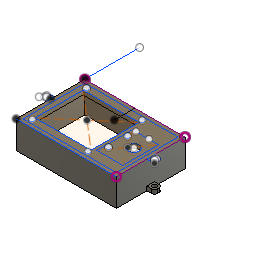
Suporte LCD Nokia 5110 e Botao de Encoder v3 (Autodesk Fusion 360 design; units mm, degrees)
Autodesk Fusion 360 part; units mm, degrees
sketch "Sketch1" plane through (0, 0, 0) normal (0, 1, 0) x (1, 0, 0)
  line L0 (72, -50) -> (-1, -50)
  line L1 (1.5, -2.5) -> (69.5, -2.5)
  line L2 (69.5, -47.5) -> (1.5, -47.5)
  circle A0 centre (5.5, -5.25) radius 1.5
  circle A1 centre (5.5, -44.75) radius 1.5
  circle A2 centre (46, -5.25) radius 1.5
  circle A3 centre (46, -44.75) radius 1.5
  line L3 (46, -7.5) -> (5.25, -7.5)
  line L4 (5.25, -7.5) -> (5.25, -42.5)
  line L5 (5.25, -42.5) -> (46, -42.5)
  line L6 (46, -42.5) -> (46, -7.5)
  line L7 (46, -7.5) -> (5.25, -42.5) construction
  line L8 (5.25, -7.5) -> (46, -42.5) construction
  line L9 (72, 0) -> (-1, 0)
  line L10 (-1, 39.9342) -> (-1, -50)
  line L11 (1.5, -47.5) -> (1.5, -2.5)
  line L12 (67.25, -14.5) -> (48.25, -14.5)
  line L13 (48.25, -14.5) -> (48.25, -40.5)
  line L14 (48.25, -40.5) -> (67.25, -40.5)
  line L15 (67.25, -40.5) -> (67.25, -14.5)
  line L16 (67.25, -14.5) -> (48.25, -40.5) construction
  line L17 (48.25, -14.5) -> (67.25, -40.5) construction
  line L18 (67.25, -14.5) -> (60.25, -14.5)
  line L19 (69.5, -2.5) -> (69.5, -47.5)
  line L20 (72, 0) -> (72, -50)
  circle A4 centre (60.25, -25.5) radius 3.875
  line L21 (48.25, -14.5) -> (50.75, -14.5)
  circle A5 centre (50.75, -20.5) radius 1.5
  circle A6 centre (50.75, -34.5) radius 1.5
  point P0 (25.625, -25)
  point P1 (57.75, -27.5)
  dimension "d10" = 3
  dimension "d12" = 35
  dimension "d15" = 19
  dimension "d19" = 26
  dimension "d20" = 2.5
  dimension "d21" = 40.75
  dimension "d22" = 4
  dimension "d30" = 7.75
  dimension "d31" = 2.5
  dimension "d32" = 6
  dimension "d34" = 3
  dimension "d35" = 3
  dimension "d36" = 7
  dimension "d37" = 11
  constraint horizontal L9
  constraint horizontal L0
  constraint perpendicular L3 L4
  constraint parallel L3 L5
  constraint parallel L4 L6
  constraint horizontal L3
  constraint coincident L7 P0
  constraint coincident L8 P0
  constraint perpendicular L9 L10
  constraint parallel L1 L9
  constraint parallel L0 L2
  constraint perpendicular L12 L13
  constraint parallel L12 L14
  constraint parallel L13 L15
  constraint horizontal L12
  constraint coincident L16 P1
  constraint coincident L17 P1
  constraint horizontal L18
  constraint coincident L9.end L10
  constraint perpendicular L13 L21
  measures "d10" diameter of A3
  measures "d12" distance of L3.end L4.end
  measures "d15" distance of L13.end L14.end
  measures "d19" distance of L12.start L14.end
  measures "d20" distance of L10 L11
  measures "d21" distance of L3.start L3.end
  measures "d22" distance of A0.centre L11
  measures "d30" diameter of A4
  measures "d31" distance of L12.end L21.end
  measures "d32" distance of L21.end A5.centre
  measures "d34" diameter of A5
  measures "d35" diameter of A6
  measures "d36" distance of L15 A4.centre
  measures "d37" distance of L12 A4.centre
extrude "Extrude1" add sketch "Sketch1" against normal blind 3 contours L1 L2 L11 L19 | L12 L13 L14 L15 L18 L21
extrude "Extrude2" add sketch "Sketch1" against normal blind 20 contours L0 L9 L10 L20
sketch "Sketch2" plane through (0, 0, 0) normal (0, 1, 0) x (1, 0, 0)
  line L0 (72, 0) -> (72, -50)
  line L1 (72, -25) -> (72, -27.75)
  line L2 (72, -27.75) -> (75.5, -27.75)
  line L3 (77.5, -25.75) -> (77.5, -24.25)
  line L4 (75.5, -22.25) -> (72, -22.25)
  line L5 (72, -22.25) -> (72, -27.75)
  circle A0 centre (74.75, -25) radius 1.5
  line L6 (72, 0) -> (-1, 0)
  line L7 (35.5, 0) -> (35.5, -15)
  arc A1 (77.5, -24.25) -> (75.5, -22.25) centre (75.5, -24.25) ccw
  arc A2 (75.5, -27.75) -> (77.5, -25.75) centre (75.5, -25.75) ccw
  circle A3 centre (-3.75, -25) radius 1.5
  arc A4 (-6.5, -25.75) -> (-4.5, -27.75) centre (-4.5, -25.75) ccw
  arc A5 (-4.5, -22.25) -> (-6.5, -24.25) centre (-4.5, -24.25) ccw
  line L8 (-1, -22.25) -> (-1, -27.75)
  line L9 (-4.5, -22.25) -> (-1, -22.25)
  line L10 (-6.5, -25.75) -> (-6.5, -24.25)
  line L11 (-1, -27.75) -> (-4.5, -27.75)
  line L12 (-1, 0) -> (-1, -50)
  line L13 (-1, -25) -> (-1, -27.75)
  point P0 (77.5, -27.75)
  point P1 (-6.5, -27.75)
  dimension "d45" = 5.5
  dimension "d46" = 5.5
  dimension "d47" = 3
  dimension "d48" = 15
  dimension "d49" = 2
  dimension "d50" = 2
  constraint midpoint L0 L1.start
  constraint horizontal L2
  constraint vertical L3
  constraint horizontal L4
  constraint vertical L5
  constraint midpoint L6 L7.start
  constraint perpendicular L6 L7
  constraint tangent L3 A1
  constraint tangent L4 A1
  constraint coincident P0 L3
  constraint coincident P0 L2
  constraint tangent L3 A2
  constraint tangent L2 A2
  constraint symmetric L0.start L7 L6.end
  constraint symmetric L0.end L7 L12.end
  constraint symmetric L1.start L7 L13.start
  constraint symmetric L1.end L7 L8.end
  constraint symmetric P0 L7 P1
  constraint symmetric L4.end L7 L8.start
  constraint symmetric A0 L7 A3
  constraint symmetric L7 L3.end A5.end
  constraint symmetric L7 L4.start A5.start
  constraint symmetric L7 A1 A5
  constraint symmetric L7 L3.start A4.start
  constraint symmetric L7 L2.end A4.end
  constraint symmetric L7 A2 A4
  measures "d45" distance of L1.end L4.end
  measures "d46" distance of L1.end P0
  measures "d47" diameter of A0
  measures "d48" distance of L7.start L7.end
  measures "d49" radius of A1
  measures "d50" radius of A2
extrude "Extrude3" add sketch "Sketch2" against normal blind 20 contours A4 A5 L8 L9 L10 L11 L12 L13
extrude "Extrude4" cut sketch "Sketch2" against normal blind 17 contours A4 A5 L8 L9 L10 L11 L12 L13
extrude "Extrude5" add sketch "Sketch2" against normal blind 20 contours L0 L1 L2 L3 L4 L5 A1 A2
extrude "Extrude6" cut sketch "Sketch2" against normal blind 17 contours L0 L1 L2 L3 L4 L5 A1 A2
